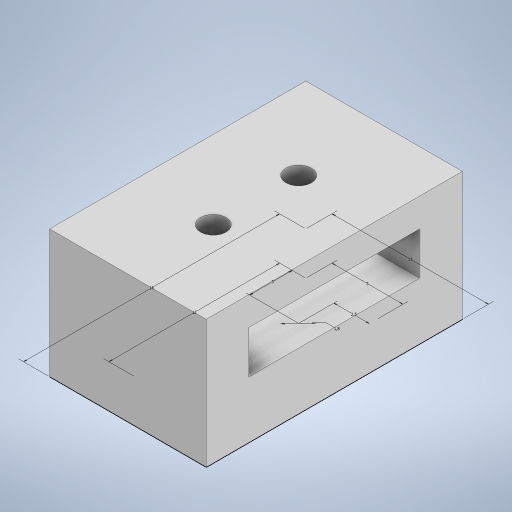
# Autodesk Inventor part: pokus
Saved by Autodesk Inventor 2024 (Build 280153000, 153)
## iProperties
Created: 2023-12-03
Part Number: pokus
Material: Všeobecné
Document SubType Name: Modeling
Designer: Roman Suk
Density: 1 g/cm^3
Appearance: Výchozí
Author: Roman Suk
MASSSFP: 400 g
SFP: 4HR
Autodesk Inventor part; units mm, degrees
ref_plane "YZ Plane" through (0, 0, 0) normal (1, 0, 0) x (0, 1, 0)
ref_plane "XZ Plane" through (0, 0, 0) normal (0, 1, 0) x (-1, 0, 0)
ref_plane "XY Plane" through (0, 0, 0) normal (0, 0, 1) x (1, 0, 0)
sketch "Sketch2" plane through (0, 0, 0) normal (0, 1, 0) x (-1, 0, 0)
  line L0 (-2.5, 6) -> (2.5, 6)
  line L1 (2.5, 6) -> (2.5, -6)
  line L2 (2.5, -6) -> (-2.5, -6)
  line L3 (-2.5, -6) -> (-2.5, 6)
  line L4 (-2.5, 6) -> (2.5, -6) construction
  line L5 (2.5, 6) -> (-2.5, -6) construction
  line L6 (-5.5, 9) -> (5.5, 9)
  line L7 (5.5, 9) -> (5.5, -9)
  line L8 (5.5, -9) -> (-5.5, -9)
  line L9 (-5.5, -9) -> (-5.5, 9)
  line L10 (-5.5, 9) -> (5.5, -9) construction
  line L11 (5.5, 9) -> (-5.5, -9) construction
  line L12 (-2.5, 0) -> (2.5, 0)
  circle A0 centre (0, -3) radius 0.9
  circle A1 centre (0, 3) radius 0.9
  point P0 (0, 0)
  dimension "d2" = 5
  dimension "d3" = 12
  dimension "d4" = 11
  dimension "d5" = 18
  dimension "d13" = 1.8
  dimension "d14" = 2.5
  dimension "d15" = 3
  constraints: 26 end point, 6 midpoint, 4 parallel, 2 centre point, 2 horizontal, 2 perpendicular, 1 symmetric about line, 1 other
  measures "d2" distance of L1.end L2.end
  measures "d3" distance of L0.end L1.end
  measures "d4" distance of L7.end L8.end
  measures "d5" distance of L6.end L7.end
  measures "d13" diameter of A0
  measures "d14" distance from line of L3 A0.centre
  measures "d15" distance from line of L2 A0.centre
extrude "Extrusion2" add sketch "Sketch2" along normal blind 4 contours L6 L7 L8 L9
sketch "Sketch3" plane through (0, 4, 0) normal (0, 1, 0) x (1, 0, 0)
  line L0 (-2.5, 6) -> (2.5, 6) projected
  line L1 (2.5, -6) -> (-2.5, -6)
  line L2 (-2.5, -6) -> (-2.5, 6)
  line L3 (-2.5, 6) -> (2.5, 6)
  line L4 (2.5, 6) -> (2.5, -6)
  line L5 (2.5, -6) -> (-2.5, 6) construction
  line L6 (-2.5, -6) -> (2.5, 6) construction
  line L7 (5.5, 9) -> (-5.5, 9)
  line L8 (-5.5, 9) -> (-5.5, -9)
  line L9 (-5.5, -9) -> (5.5, -9)
  line L10 (5.5, -9) -> (5.5, 9)
  line L11 (5.5, 9) -> (-5.5, -9) construction
  line L12 (-5.5, 9) -> (5.5, -9) construction
  line L13 (2.5, -6) -> (5.5, -6)
  line L14 (2.5, 6) -> (5.5, 6)
  point P0 (0, 0)
  constraints: 28 end point, 4 midpoint, 4 parallel, 3 perpendicular, 3 point on line, 2 horizontal
extrude "Extrusion3" add sketch "Sketch3" along normal blind 3 contours L2 L1 L13 L10 L9 L8 L7 L14 L0
sketch "Sketch4" plane through (0, 7, 0) normal (0, 1, 0) x (1, 0, 0)
  line L0 (5.5, 9) -> (-5.5, 9) projected
  line L1 (5.5, -9) -> (-5.5, -9)
  line L2 (-5.5, -9) -> (-5.5, 9)
  line L3 (-5.5, 9) -> (5.5, 9)
  line L4 (5.5, 9) -> (5.5, -9)
  line L5 (5.5, -9) -> (-5.5, 9) construction
  line L6 (-5.5, -9) -> (5.5, 9) construction
  point P0 (0, 0)
  constraints: 12 end point, 2 midpoint, 2 parallel, 1 horizontal, 1 perpendicular
extrude "Extrusion4" add sketch "Sketch4" along normal blind 2
extrude "Extrusion5" cut sketch "Sketch2" along normal through all contours A0 | A1
body "Solid2"
